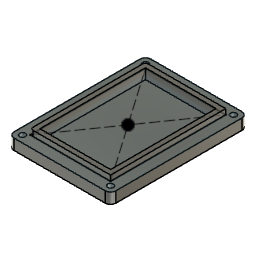
Read-Write Enclosure Lid v1 (Autodesk Fusion 360 design; units mm, degrees)
Autodesk Fusion 360 part; units mm, degrees
sketch "Sketch1" plane through (0, 0, 0) normal (0, 0, 1) x (1, 0, 0)
  line L0 (47.5, 63.75) -> (-47.5, 63.75)
  line L1 (-47.5, 63.75) -> (-47.5, -63.75)
  line L2 (-47.5, -63.75) -> (47.5, -63.75)
  line L3 (47.5, -63.75) -> (47.5, 63.75)
  line L4 (47.5, 63.75) -> (-47.5, -63.75) construction
  line L5 (-47.5, 63.75) -> (47.5, -63.75) construction
  dimension "d1" = 95
  dimension "d2" = 127.5
  constraint horizontal L0
  constraint perpendicular L0 L1
  constraint parallel L0 L2
  constraint parallel L1 L3
  constraint coincident L4 origin
  constraint coincident L5 origin
  measures "d1" distance of L1.end L2.end
  measures "d2" distance of L0.end L1.end
extrude "Extrude1" add sketch "Sketch1" along normal blind 10
fillet "Fillet1" radius 5 1 edges at (47.5, -63.75, 5)
fillet "Fillet2" radius 5 1 edges at (47.5, 63.75, 5)
fillet "Fillet3" radius 5 1 edges at (-47.5, 63.75, 5)
fillet "Fillet4" radius 5 1 edges at (-47.5, -63.75, 5)
hole "Hole17" at (41, -57.25, 10) direction (0, 0, -1) diameter 5.5 depth 5 tip angle 180
hole "Hole18" at (-41, -57.25, 10) direction (0, 0, -1) diameter 5.5 depth 5 tip angle 180
hole "Hole19" at (-41, 57.25, 10) direction (0, 0, -1) diameter 5.5 depth 5 tip angle 180
hole "Hole20" at (41, 57.25, 10) direction (0, 0, -1) diameter 5.5 depth 5 tip angle 180
sketch "Sketch77" plane through (0, 0, 10) normal (0, 0, 1) x (-1, 0, 0)
  circle A0 centre (-41, -57.25) radius 2.75
  circle A1 centre (41, -57.25) radius 2.75
  circle A2 centre (41, 57.25) radius 2.75
  circle A3 centre (-41, 57.25) radius 2.75
  arc A4 (47.5, 58.75) -> (42.5, 63.75) centre (42.5, 58.75) ccw
  line L0 (42.5, 63.75) -> (-42.5, 63.75)
  arc A5 (-42.5, 63.75) -> (-47.5, 58.75) centre (-42.5, 58.75) ccw
  line L1 (-47.5, 58.75) -> (-47.5, -58.75)
  arc A6 (-47.5, -58.75) -> (-42.5, -63.75) centre (-42.5, -58.75) ccw
  line L2 (-42.5, -63.75) -> (42.5, -63.75)
  arc A7 (42.5, -63.75) -> (47.5, -58.75) centre (42.5, -58.75) ccw
  line L3 (47.5, -58.75) -> (47.5, 58.75)
  line L4 (-37.4, 53.65) -> (37.4, 53.65)
  line L5 (37.4, 53.65) -> (37.4, -53.65)
  line L6 (37.4, -53.65) -> (-37.4, -53.65)
  line L7 (-37.4, -53.65) -> (-37.4, 53.65)
  line L8 (-37.4, 53.65) -> (37.4, -53.65) construction
  line L9 (37.4, 53.65) -> (-37.4, -53.65) construction
  dimension "d279" = 74.8
  dimension "d280" = 107.3
  constraint horizontal L4
  constraint perpendicular L4 L5
  constraint parallel L4 L6
  constraint parallel L5 L7
  constraint coincident L8 origin
  constraint coincident L9 origin
  measures "d279" distance of L5.end L6.end
  measures "d280" distance of L4.end L5.end
sketch "Sketch78" plane through (0, 0, 0) normal (0, 0, -1) x (1, 0, 0)
  arc A0 (-42.5, 63.75) -> (-47.5, 58.75) centre (-42.5, 58.75) ccw
  line L0 (-47.5, 58.75) -> (-47.5, -58.75)
  arc A1 (-47.5, -58.75) -> (-42.5, -63.75) centre (-42.5, -58.75) ccw
  line L1 (-42.5, -63.75) -> (42.5, -63.75)
  arc A2 (42.5, -63.75) -> (47.5, -58.75) centre (42.5, -58.75) ccw
  line L2 (47.5, -58.75) -> (47.5, 58.75)
  arc A3 (47.5, 58.75) -> (42.5, 63.75) centre (42.5, 58.75) ccw
  line L3 (42.5, 63.75) -> (-42.5, 63.75)
  line L4 (45.5964, -58.112) -> (44.0447, -53.7004)
  line L5 (44.0447, -53.7004) -> (39.4483, -52.8384)
  line L6 (39.4483, -52.8384) -> (36.4036, -56.388)
  line L7 (36.4036, -56.388) -> (37.9553, -60.7996)
  line L8 (37.9553, -60.7996) -> (42.5517, -61.6616)
  line L9 (42.5517, -61.6616) -> (45.5964, -58.112)
  line L10 (-42.2713, -61.7504) -> (-37.7382, -60.6012)
  line L11 (-37.7382, -60.6012) -> (-36.4669, -56.1008)
  line L12 (-36.4669, -56.1008) -> (-39.7287, -52.7496)
  line L13 (-39.7287, -52.7496) -> (-44.2618, -53.8988)
  line L14 (-44.2618, -53.8988) -> (-45.5331, -58.3992)
  line L15 (-45.5331, -58.3992) -> (-42.2713, -61.7504)
  line L16 (42.185, 61.7739) -> (37.6747, 60.5382)
  line L17 (37.6747, 60.5382) -> (36.4897, 56.0143)
  line L18 (36.4897, 56.0143) -> (39.815, 52.7261)
  line L19 (39.815, 52.7261) -> (44.3253, 53.9618)
  line L20 (44.3253, 53.9618) -> (45.5103, 58.4857)
  line L21 (45.5103, 58.4857) -> (42.185, 61.7739)
  line L22 (-45.4838, 58.5789) -> (-44.3927, 54.0314)
  line L23 (-44.3927, 54.0314) -> (-39.909, 52.7025)
  line L24 (-39.909, 52.7025) -> (-36.5162, 55.9211)
  line L25 (-36.5162, 55.9211) -> (-37.6073, 60.4686)
  line L26 (-37.6073, 60.4686) -> (-42.091, 61.7975)
  line L27 (-42.091, 61.7975) -> (-45.4838, 58.5789)
  point P0 (41, -57.25)
  point P1 (-41, -57.25)
  point P2 (41, 57.25)
  point P3 (-41, 57.25)
  dimension "d290" = 4.05
  dimension "d291" = 4.05
  dimension "d292" = 4.05
  dimension "d293" = 4.05
  measures "d290" distance of P0 L9
  measures "d291" distance of P1 L15
  measures "d292" distance of P2 L21
  measures "d293" distance of P3 L27
extrude "Extrude4" add sketch "Sketch77" along normal blind 5 contours L4 L5 L6 L7
fillet "Fillet13" radius 2.5 2 edges at (-37.4, 53.65, 12.5) (-37.4, -53.65, 12.5)
shell "Shell3" thickness 4.5 removed faces 1 at (12.4667, -17.05, 15)
extrude "Extrude5" cut sketch "Sketch78" against normal blind 5 contours L4 L5 L6 L7 L8 L9 | L10 L11 L12 L13 L14 L15 | L16 L17 L18 L19 L20 L21 | L22 L23 L24 L25 L26 L27
